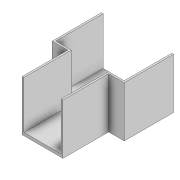
# Autodesk Inventor part: large_room1
Saved by Autodesk Inventor 2021 (Build 250183000, 183)
## iProperties
Created: 2022-05-19
Part Number: large_room1
Material: Generic
Document SubType Name: Modeling
Designer: Derm
Density: 1 g/cm^3
Appearance: Default
Author: Derm
Autodesk Inventor part; units mm, degrees
ref_plane "YZ Plane" through (0, 0, 0) normal (1, 0, 0) x (0, 1, 0)
ref_plane "XZ Plane" through (0, 0, 0) normal (0, 1, 0) x (-1, 0, 0)
ref_plane "XY Plane" through (0, 0, 0) normal (0, 0, 1) x (1, 0, 0)
sketch "Sketch1" plane through (0, 0, 0) normal (0, 1, 0) x (-1, 0, 0)
  line L0 (0, 0) -> (0, -14.0125) construction
  line L1 (9.9647, 25.4) -> (9.9647, 0)
  line L2 (9.9647, 0) -> (18.3253, 0)
  line L3 (18.3253, 0) -> (18.3253, -25.4)
  line L4 (10.9285, 25.4) -> (10.9285, 0.9638)
  line L5 (10.9285, 0.9638) -> (19.2891, 0.9638)
  line L6 (19.2891, 0.9638) -> (19.2891, -25.4)
  line L7 (10.9285, 25.4) -> (9.9647, 25.4)
  line L8 (18.3253, -25.4) -> (19.2891, -25.4)
  line L9 (-9.9647, 25.4) -> (-9.9647, 0)
  line L10 (-9.9647, 0) -> (-18.3253, 0)
  line L11 (-18.3253, 0) -> (-18.3253, -25.4)
  line L12 (-10.9285, 25.4) -> (-10.9285, 0.9638)
  line L13 (-10.9285, 0.9638) -> (-19.2891, 0.9638)
  line L14 (-19.2891, 0.9638) -> (-19.2891, -25.4)
  line L15 (-10.9285, 25.4) -> (-9.9647, 25.4)
  line L16 (-18.3253, -25.4) -> (-19.2891, -25.4)
  dimension "d4" = 25.4
  dimension "d5" = 25.4
  constraints: 34 end point, 8 symmetric about line, 4 perpendicular, 2 horizontal, 2 vertical, 2 other
  measures "d4" distance between parallel lines of L8 L2
  measures "d5" distance between parallel lines of L2 L7
extrude "Extrusion1" add sketch "Sketch1" against normal mid plane 25.4
sketch "Sketch2" plane through (0, -12.7, 0) normal (0, -1, 0) x (1, 0, 0)
  line L0 (-9.9647, 0) -> (-9.9647, 25.4) projected
  line L1 (-9.9647, 25.4) -> (-10.9285, 25.4) projected
  line L2 (-10.9285, 25.4) -> (-10.9285, 0.9638) projected
  line L3 (-10.9285, 0.9638) -> (-19.2891, 0.9638) projected
  line L4 (-19.2891, 0.9638) -> (-19.2891, -25.4) projected
  line L5 (-19.2891, -25.4) -> (-18.3253, -25.4) projected
  line L6 (-18.3253, -25.4) -> (-18.3253, 0) projected
  line L7 (-18.3253, 0) -> (-9.9647, 0) projected
  line L8 (19.2891, 0.9638) -> (10.9285, 0.9638) projected
  line L9 (10.9285, 0.9638) -> (10.9285, 25.4) projected
  line L10 (10.9285, 25.4) -> (9.9647, 25.4) projected
  line L11 (9.9647, 25.4) -> (9.9647, 0) projected
  line L12 (9.9647, 0) -> (18.3253, 0) projected
  line L13 (18.3253, 0) -> (18.3253, -25.4) projected
  line L14 (18.3253, -25.4) -> (19.2891, -25.4) projected
  line L15 (19.2891, -25.4) -> (19.2891, 0.9638) projected
  line L16 (10.9285, 25.4) -> (9.9647, 25.4) projected
  line L17 (-9.9647, 25.4) -> (-10.9285, 25.4) projected
  line L18 (10.9285, 25.4) -> (-10.9285, 25.4)
  line L19 (19.2891, 0.9638) -> (19.2891, -25.4) projected
  line L20 (19.2891, -25.4) -> (-19.2891, -25.4)
  point P0 (0, 0)
  constraints: 4 end point, 1 horizontal, 1 perpendicular
extrude "Extrusion2" add sketch "Sketch2" along normal blind 1.5875
body "Solid1"
